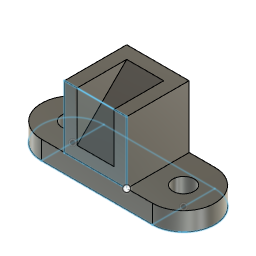
Model 2 v1 (Autodesk Fusion 360 design; units mm, degrees)
Autodesk Fusion 360 part; units mm, degrees
note: some values were not read from the file. Set by a fixed rule: which face or edge a step refers to.
sketch "Sketch1" plane through (0, 0, 0) normal (0, 0, 1) x (1, 0, 0)
  line L0 (0, 64.3011) -> (114, 64.3011)
  line L1 (114, 64.3011) -> (114, 0.3011)
  line L2 (114, 0.3011) -> (0, 0.3011)
  line L3 (0, 0.3011) -> (0, 64.3011)
  arc A0 (114, 0.3011) -> (114, 64.3011) centre (114, 32.3011) ccw
  arc A1 (0, 64.3011) -> (0, 0.3011) centre (0, 32.3011) ccw
  dimension "d1" = 114
  dimension "d2" = 64
  dimension "d3" = 64
  dimension "d4" = 64
  constraint horizontal L0
  constraint vertical L1
  constraint horizontal L2
  constraint vertical L3
  constraint midpoint L1 A0.centre
  constraint midpoint L3 A1.centre
  measures "d1" distance of L0.start L0.end
  measures "d2" distance of L0.start L2.end
  measures "d3" diameter of A0
  measures "d4" diameter of A1
extrude "Extrude1" add sketch "Sketch1" along normal blind 19 contours L1 A0 makes body 1
extrude "Extrude2" add sketch "Sketch1" along normal blind 19 contours L0 L1 L2 L3 | L3 A1 bodies 1
hole "Hole1" at (113.8612, 32.3859, 19) direction (0, 0, -1) diameter 22 depth 22 tip angle 118 bodies 1
hole "Hole2" at (-0.1649, 32.3354, 19) direction (0, 0, -1) diameter 22 depth 22 tip angle 180 bodies 1
sketch "Sketch2" plane through (0, 0, 0) normal (0, 1, 0) x (1, 0, 0)
  line L0 (23.8188, -19.102) -> (87.8188, -19.102)
  line L1 (87.8188, -19.102) -> (87.8188, -83.102)
  line L2 (87.8188, -83.102) -> (23.8188, -83.102)
  line L3 (23.8188, -83.102) -> (23.8188, -19.102)
  dimension "d16" = 64
  constraint horizontal L0
  constraint vertical L1
  constraint horizontal L2
  constraint vertical L3
  measures "d16" distance of L0.start L2.end
extrude "Extrude3" add sketch "Sketch2" along normal blind 64 separate body makes body 2
move_face "MoveFace1" by (0, 1, 0) 1 faces at (87.8188, 21.3333, 40.4353) on bodies 2
shell "Shell1" thickness 13 removed faces 2 at (66.4855, 21.3333, 83.102) at (45.1521, 0, 40.4353) on bodies 2
draft "Draft1" angle -45 neutral plane through (0, 0, 0) pull (0, 1, 0) 1 faces at (49.4855, 34, 32.102) on bodies 2
